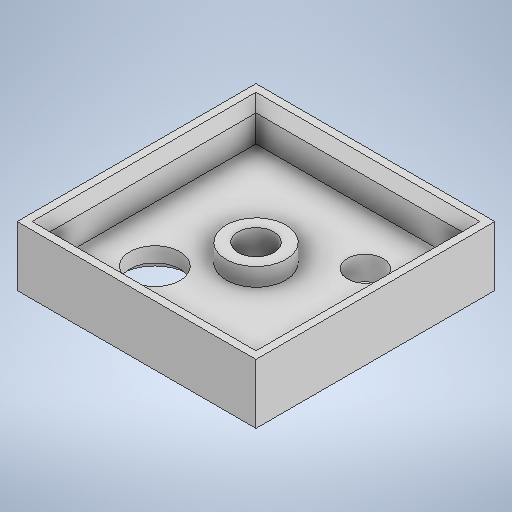
# Autodesk Inventor part: BambuLabVolcanoNozzle_silicon_innerpart2_deckel
Saved by Autodesk Inventor 2025.2 (Build 292293000, 293)
## iProperties
Created: 2025-02-18
Part Number: BambuLabVolcanoNozzle_silicon_innerpart2_deckel
Material: Generisch
Document SubType Name: Modeling
Designer: FrankFlorian
Density: 1 g/cm^3
Appearance: Vorgabe
Author: FrankFlorian
Autodesk Inventor part; units mm, degrees
ref_plane "YZ Plane" through (0, 0, 0) normal (1, 0, 0) x (0, 1, 0)
ref_plane "XZ Plane" through (0, 0, 0) normal (0, 1, 0) x (-1, 0, 0)
ref_plane "XY Plane" through (0, 0, 0) normal (0, 0, 1) x (1, 0, 0)
sketch "Skizze1" plane through (0, 0, 0) normal (0, 0, 1) x (1, 0, 0)
  line L0 (-9, 9) -> (9, 9)
  line L1 (9, 9) -> (9, -9)
  line L2 (9, -9) -> (-9, -9)
  line L3 (-9, -9) -> (-9, 9)
  line L4 (-9, 9) -> (9, -9) construction
  line L5 (9, 9) -> (-9, -9) construction
  point P0 (0, 0)
  dimension "d0" = 18
  dimension "d1" = 18
  constraints: 12 end point, 2 midpoint, 2 parallel, 1 horizontal, 1 perpendicular
  measures "d0" distance of L1.end L2.end
  measures "d1" distance of L0.end L1.end
extrude "Extrusion1" add sketch "Skizze1" along normal blind 2
sketch "Skizze2" plane through (0, 0, 2) normal (0, 0, 1) x (1, 0, 0)
  circle A0 centre (0, 0) radius 2.5
  dimension "d4" = 5
  constraints: 1 centre point, 1 coincident
  measures "d4" diameter of A0
extrude "Extrusion2" add sketch "Skizze2" along normal blind 1.5
sketch "Skizze3" plane through (0, 0, 2) normal (0, 0, 1) x (1, 0, 0)
  circle A0 centre (5, 4.1533) radius 1.5
  circle A1 centre (-4, -4.4721) radius 2.1
  line L0 (9, -9) -> (9, 9) projected
  point P0 (0, 0)
  dimension "d7" = 3
  dimension "d8" = 4.2
  dimension "d9" = 6.5
  dimension "d40" = 6
  dimension "d41" = 13
  dimension "d42" = 4
  constraints: 2 centre point
  measures "d7" diameter of A0
  measures "d8" diameter of A1
  measures "d9" distance of point (0, 0) A0.centre
  measures "d40" distance of point (0, 0) A1.centre
  measures "d41" distance from line of L0 A1.centre
  measures "d42" distance from line of L0 A0.centre
extrude "Extrusion3" cut sketch "Skizze3" against normal blind 5.25
sketch "Skizze4" plane through (0, 0, 3.5) normal (0, 0, 1) x (1, 0, 0)
  circle A0 centre (0, 0) radius 1.5
  dimension "d12" = 3
  constraints: 1 centre point, 1 coincident
  measures "d12" diameter of A0
extrude "Extrusion4" cut sketch "Skizze4" against normal blind 9
sketch "Skizze8" plane through (0, 0, 0) normal (0, 0, -1) x (-1, 0, 0)
  line L0 (-9, -9) -> (-9, 9) projected
  line L1 (9, -9) -> (-9, -9) projected
  line L2 (-9, 9) -> (9, 9)
  line L3 (9, 9) -> (9, -9)
  line L4 (9, -9) -> (-9, -9)
  line L5 (-9, -9) -> (-9, 9)
  line L6 (10, 10) -> (-10, 10)
  line L7 (-10, 10) -> (-10, -10)
  line L8 (-10, -10) -> (10, -10)
  line L9 (10, -10) -> (10, 10)
  line L10 (-8.625, 8.625) -> (8.625, 8.625)
  line L11 (8.625, 8.625) -> (8.625, -8.625)
  line L12 (8.625, -8.625) -> (-8.625, -8.625)
  line L13 (-8.625, -8.625) -> (-8.625, 8.625)
  line L14 (-8.625, 8.625) -> (8.625, -8.625) construction
  line L15 (8.625, 8.625) -> (-8.625, -8.625) construction
  point P0 (0, 0)
  dimension "d28" = 20
  dimension "d29" = 20
  dimension "d30" = 17.25
  dimension "d31" = 17.25
  constraints: 28 end point, 6 parallel, 3 horizontal, 3 perpendicular, 2 midpoint
  measures "d28" distance of L8.end L7.end
  measures "d29" distance of L7.end L6.end
  measures "d30" distance of L11.end L12.end
  measures "d31" distance of L10.end L11.end
extrude "Extrusion6" add sketch "Skizze8" against normal blind 5 contours L0 L2 L3 L1 | L9 L8 L7 L6
chamfer "Fasen2" distance 0.75 angle 45 1 edges at (-6.1, -4.4721, 0)
chamfer "Fasen3" distance 0.75 angle 45 4 edges at (0, 8.625, 5) (-8.625, 0, 5) (0, -8.625, 5) (8.625, 0, 5)
